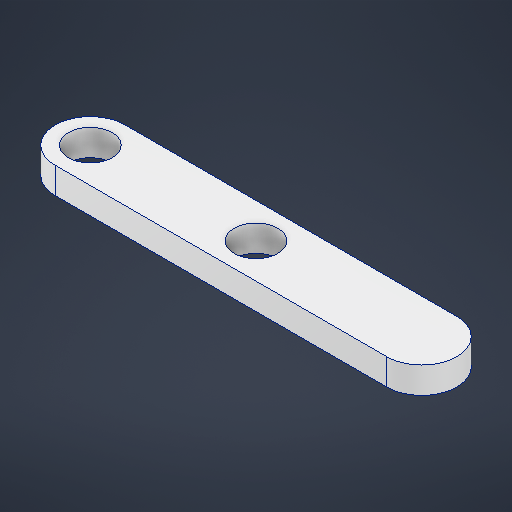
# Autodesk Inventor part: CNC-011-XAxisHardStop
Saved by Autodesk Inventor 2026.2 (Build 302298000, 298)
## iProperties
Created: 2026-06-17
Part Number: CNC-011-XAxisHardStop
Material: Aluminum 6061
Document SubType Name: Modeling
Designer: Kenji
Density: 2.7 g/cm^3
Appearance: Aluminum - Flat
Author: Kenji
Autodesk Inventor part; units mm, degrees
ref_plane "YZ Plane" through (0, 0, 0) normal (1, 0, 0) x (0, 1, 0)
ref_plane "XZ Plane" through (0, 0, 0) normal (0, 1, 0) x (-1, 0, 0)
ref_plane "XY Plane" through (0, 0, 0) normal (0, 0, 1) x (1, 0, 0)
sketch "Sketch1" plane through (0, 0, 0) normal (0, 1, 0) x (-1, 0, 0)
  circle A0 centre (0, 0) radius 2.63
  line L0 (0, 0) -> (-2.63, 0) construction
  circle A1 centre (-20, 0) radius 2.63
  circle A2 centre (0, 0) radius 4.2175 construction
  circle A3 centre (-20, 0) radius 4.2175 construction
  line L1 (0, 4.2175) -> (-40, 4.2175)
  line L2 (0, -4.2175) -> (-40, -4.2175)
  arc A4 (-40, 4.2175) -> (-40, -4.2175) centre (-40, 0) ccw
  arc A5 (0, -4.2175) -> (0, 4.2175) centre (0, 0) ccw
  dimension "d0" = 5.26
  dimension "d1" = 20
  dimension "d2" = 1.5875
  dimension "d3" = 20
  constraints: 6 end point, 6 point on circle, 5 centre point, 5 tangent, 3 horizontal, 2 coincident, 1 equal radius, 1 horizontal alignment, 1 point on line, 3 other
  measures "d1" distance of A1.centre point (0, 0)
  measures "d3" distance of A4.centre A1.centre
extrude "Extrusion1" add sketch "Sketch1" along normal blind 3.175
body "Solid1"
